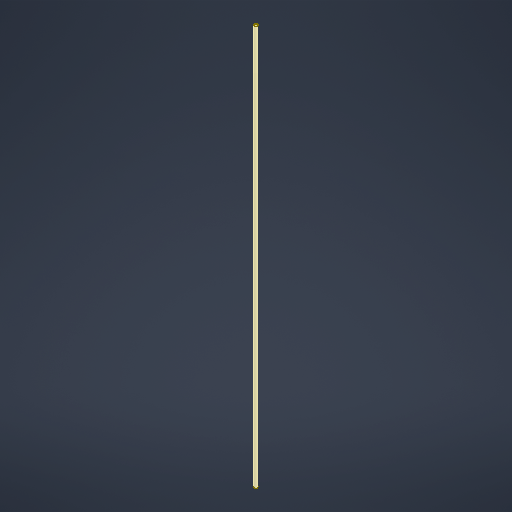
# Autodesk Inventor part: Loft Support
Saved by Autodesk Inventor 2026 (Build 300175000, 175)
## iProperties
Created: 2025-11-05
Part Number: Loft Support
Material: Nylon 6/6
Document SubType Name: Modeling
Designer: Brandon Portillo
Density: 1.13 g/cm^3
Appearance: Nylon 6
Mass: 35.4645 g
Surface Area: 628.256 cm^2
Volume: 31.3845 cm^3
Author: Brandon Portillo
Autodesk Inventor part; units mm, degrees
ref_plane "YZ Plane" through (0, 0, 0) normal (1, 0, 0) x (0, 1, 0)
ref_plane "XZ Plane" through (0, 0, 0) normal (0, 1, 0) x (-1, 0, 0)
ref_plane "XY Plane" through (0, 0, 0) normal (0, 0, 1) x (1, 0, 0)
sketch "Sketch1" plane through (0, 0, 0) normal (0, 1, 0) x (-1, 0, 0)
  circle A0 centre (0, 0) radius 5
  dimension "d0" = 10
  constraints: 1 centre point, 1 coincident
  measures "d0" diameter of A0
extrude "Extrusion1" add sketch "Sketch1" along normal blind 1110
shell "Shell1" thickness 1 removed faces 2 at (0.591, 1110, 1.5584) at (0.591, 0, 1.5584)
body "Solid1"
